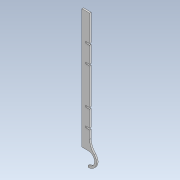
# Autodesk Inventor part: chassis_1_5
Saved by Autodesk Inventor 2022 (Build 260153000, 153)
## iProperties
Created: 2023-04-28
Part Number: chassis_1_5
Material: 一般
Document SubType Name: Modeling
Designer: Johnny Jou
Density: 1 g/cm^3
Appearance: 預設
Author: Johnny Jou
Autodesk Inventor part; units mm, degrees
ref_plane "YZ Plane" through (0, 0, 0) normal (1, 0, 0) x (0, 1, 0)
ref_plane "XZ Plane" through (0, 0, 0) normal (0, 1, 0) x (-1, 0, 0)
ref_plane "XY Plane" through (0, 0, 0) normal (0, 0, 1) x (1, 0, 0)
sketch "草圖1" plane through (0, 0, 0) normal (0, 0, 1) x (1, 0, 0)
  arc A0 (-7.5, 147.4544) -> (-7.5, 136.5456) centre (-10, 142) ccw construction
  arc A1 (-10, 4.5) -> (1.3043, 31.8231) centre (-10, 20.5) ccw
  line L0 (-10, 20.5) -> (-10, 4.5) construction
  line L1 (-10, 20.5) -> (-10, 48.1702) construction
  line L2 (-10, 8.3) -> (-10, 4.5)
  line L3 (-7.5, 266.3035) -> (-22.5, 266.3035)
  line L4 (-22.5, 266.3035) -> (-22.5, 48.1702)
  line L5 (-22.5, 48.1702) -> (-10, 48.1702) construction
  line L6 (-7.5, 36.5) -> (-7.5, 53.0538) construction
  line L7 (-7.5, 36.5) -> (-7.5, 36.3035) construction
  line L8 (-10, 48.1702) -> (-10, 32.7) construction
  line L9 (-10, 32.7) -> (-22.5, 32.7)
  line L10 (-22.5, 32.7) -> (-22.5, 48.1702)
  arc A2 (-7.5, 53.0538) -> (1.3043, 31.8231) centre (22.5, 53.0538) ccw
  arc A3 (1.3043, 31.8231) -> (-7.5, 36.3035) centre (-10, 20.5) ccw construction
  line L11 (-7.5, 53.0538) -> (-7.5, 69.05)
  line L12 (-7.5, 214.95) -> (-15, 214.95)
  line L13 (-15, 214.95) -> (-15, 212)
  line L14 (-15, 212) -> (-7.5, 212)
  line L15 (-7.5, 212) -> (-7.5, 214.95) construction
  line L16 (-7.5, 179.95) -> (-15, 179.95)
  line L17 (-15, 179.95) -> (-15, 177)
  line L18 (-15, 177) -> (-7.5, 177)
  line L19 (-7.5, 177) -> (-7.5, 179.95) construction
  line L20 (-7.5, 107) -> (-15, 107)
  line L21 (-15, 107) -> (-15, 104.05)
  line L22 (-15, 104.05) -> (-7.5, 104.05)
  line L23 (-7.5, 104.05) -> (-7.5, 107) construction
  line L24 (-7.5, 72) -> (-15, 72)
  line L25 (-15, 72) -> (-15, 69.05)
  line L26 (-15, 69.05) -> (-7.5, 69.05)
  line L27 (-7.5, 69.05) -> (-7.5, 72) construction
  line L28 (-7.5, 212) -> (-7.5, 214.95) construction
  line L29 (-7.5, 179.95) -> (-7.5, 212)
  line L30 (-7.5, 177) -> (-7.5, 179.95) construction
  line L31 (-7.5, 107) -> (-7.5, 177)
  line L32 (-7.5, 104.05) -> (-7.5, 107) construction
  line L33 (-7.5, 72) -> (-7.5, 104.05)
  line L34 (-7.5, 69.05) -> (-7.5, 72) construction
  line L35 (-7.5, 214.95) -> (-7.5, 266.3035)
  arc A4 (-10, 8.3) -> (-10, 32.7) centre (-10, 20.5) ccw
  arc A5 (-12.7221, 32.7) -> (-10, 8) centre (-10, 20.5) ccw construction
  point P0 (0, 0)
  dimension "d12" = 16
  dimension "d13" = 180
  dimension "d14" = 15
  dimension "d16" = 60
  dimension "d17" = 35
  dimension "d18" = 70
  dimension "d19" = 35
  dimension "d20" = 70
  dimension "d21" = 2.95
  dimension "d22" = 2.95
  dimension "d23" = 2.95
  dimension "d24" = 2.95
  dimension "d25" = 7.5
  dimension "d26" = 230
  dimension "d30" = 24.4
  dimension "d31" = 25
  constraints: 72 end point, 18 parallel, 12 point on circle, 12 tangent, 11 point on line, 7 perpendicular, 6 centre point, 6 horizontal, 2 coincident, 2 collinear, 1 vertical, 3 other
  measures "d12" radius of A1
  measures "d13" angle of L0 L1
  measures "d14" distance between parallel lines of L4 L6
  measures "d16" diameter of A2
  measures "d17" distance from line of L20 A0.centre
  measures "d18" distance from line of L24 A0.centre
  measures "d19" distance from line of L18 A0.centre
  measures "d20" distance from line of L14 A0.centre
  measures "d21" distance of L16.end L17.end
  measures "d22" distance of L12.end L13.end
  measures "d23" distance of L20.end L21.end
  measures "d24" distance of L24.end L25.end
  measures "d25" distance between parallel lines of L11 L25
  measures "d26" distance from line of L7.end L3
  measures "d30" diameter of A4
  measures "d31" diameter of A5
extrude "擠出1" add sketch "草圖1" along normal blind 3
equation "\"d25\" = 0.5 * d14"
